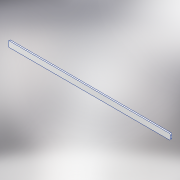
# Autodesk Inventor part: 2021-01-008
Saved by Autodesk Inventor 2020.2 (Build 242310000, 310)
## iProperties
Created: 2020-10-08
Part Number: 2021-01-008
Material: Aluminum 6061
Document SubType Name: Modeling
Designer: carso
Density: 2.7 g/cm^3
Appearance: Aluminum - Flat
Mass: 37.4495 g
Surface Area: 115.086 cm^2
Volume: 13.8702 cm^3
Author: carso
Autodesk Inventor part; units mm, degrees
ref_plane "YZ Plane" through (0, 0, 0) normal (1, 0, 0) x (0, 1, 0)
ref_plane "XZ Plane" through (0, 0, 0) normal (0, 1, 0) x (-1, 0, 0)
ref_plane "XY Plane" through (0, 0, 0) normal (0, 0, 1) x (1, 0, 0)
sketch "Sketch1" plane through (0, 0, 0) normal (0, 0, 1) x (1, 0, 0)
  line L0 (0, -3) -> (349.95, -3)
  line L1 (352.95, -6) -> (352.95, -13.05)
  line L2 (349.95, -16.05) -> (0, -16.05)
  line L3 (-3, -13.05) -> (-3, -6)
  arc A0 (352.95, -6) -> (349.95, -3) centre (349.95, -6) ccw
  arc A1 (349.95, -16.05) -> (352.95, -13.05) centre (349.95, -13.05) ccw
  arc A2 (0, -3) -> (-3, -6) centre (0, -6) ccw
  arc A3 (-3, -13.05) -> (0, -16.05) centre (0, -13.05) ccw
  point P0 (0, 0)
  point P1 (-6, -19.05)
  dimension "d0" = 3
  constraints: 8 end point, 8 point on circle, 8 tangent, 4 centre point, 3 equal radius, 2 parallel, 1 horizontal, 1 perpendicular
  measures "d0" radius of A0
extrude "Extrusion1" add sketch "Sketch1" along normal blind 3
sketch "Sketch2" plane through (0, 0, 3) normal (0, 0, 1) x (1, 0, 0)
  line L0 (-3, -3) -> (352.95, -3)
  line L1 (352.95, -3) -> (352.95, -16.05)
  line L2 (352.95, -16.05) -> (-3, -16.05)
  line L3 (-3, -16.05) -> (-3, -3)
  line L4 (174.975, -9.525) -> (174.975, -13.6338)
  line L5 (33.6, -9.525) -> (316.35, -9.525) construction
  line L6 (33.6, -11.025) -> (316.35, -11.025)
  line L7 (316.35, -8.025) -> (33.6, -8.025)
  arc A0 (33.6, -8.025) -> (33.6, -11.025) centre (33.6, -9.525) ccw
  arc A1 (316.35, -11.025) -> (316.35, -8.025) centre (316.35, -9.525) ccw
  point P0 (0, 0)
  dimension "d4" = 3
  constraints: 18 end point, 4 point on circle, 4 tangent, 3 parallel, 2 centre point, 2 perpendicular, 1 horizontal, 1 midpoint, 1 vertical
  measures "d4" diameter of A1
sketch "Sketch3" plane through (0, 0, 0) normal (0, 0, -1) x (-1, 0, 0)
  line L0 (-352.95, -3) -> (3, -3)
  line L1 (3, -3) -> (3, -16.05)
  line L2 (3, -16.05) -> (-352.95, -16.05)
  line L3 (-352.95, -16.05) -> (-352.95, -3)
  line L4 (0, -16.05) -> (-349.95, -16.05)
  line L5 (-352.95, -3) -> (-322.95, -3)
  line L6 (-322.95, -3) -> (-322.95, -16.05)
  line L7 (-322.95, -16.05) -> (-352.95, -16.05)
  line L8 (-352.95, -16.05) -> (-352.95, -3)
  line L9 (3, -3) -> (-27, -3)
  line L10 (-27, -3) -> (-27, -16.05)
  line L11 (-27, -16.05) -> (3, -16.05)
  line L12 (3, -16.05) -> (3, -3)
  line L13 (-322.95, -3) -> (-322.95, -9.525)
  line L14 (-322.95, -9.525) -> (-27, -9.525)
  line L15 (-322.95, -9.525) -> (-292.95, -9.525)
  line L16 (-27, -9.525) -> (-57, -9.525)
  circle A0 centre (-292.95, -9.525) radius 2.5
  circle A1 centre (-57, -9.525) radius 2.5
  line L17 (-290.45, -9.525) -> (-285.45, -9.525)
  line L18 (-352.95, -3) -> (3, -3)
  line L19 (3, -3) -> (3, -16.05)
  line L20 (3, -16.05) -> (-352.95, -16.05)
  line L21 (-352.95, -16.05) -> (-352.95, -3)
  point P0 (0, 0)
  point P1 (-355.95, -19.05)
  dimension "d7" = 30
  dimension "d8" = 30
  dimension "d9" = 6.525
  dimension "d10" = 30
  dimension "d11" = 30
  dimension "d12" = 5
  dimension "d13" = 5
  constraints: 44 end point, 8 parallel, 6 point on line, 4 horizontal, 4 perpendicular, 2 coincident, 2 midpoint, 1 centre point, 1 horizontal alignment, 2 other
  measures "d7" distance of L6.end L7.end
  measures "d8" distance of L11.end L10.end
  measures "d9" distance of L5.end L13.end
  measures "d10" distance of L13.end L15.end
  measures "d11" distance of L14.end L16.end
  measures "d12" diameter of A1
  measures "d13" distance of L17.start L17.end
extrude "Extrusion3" cut sketch "Sketch3" against normal blind 1 contours A0 L14 | L14 A0 | A1 L14 | L14 A1
sketch "Sketch4" plane through (57, -9.525, 1) normal (0, 0, -1) x (-1, 0, 0)
  circle A0 centre (0, 0) radius 2.5
  circle A1 centre (-235.95, 0) radius 2.5 projected
  circle A2 centre (-235.95, 0) radius 2.5
  circle A3 centre (-235.95, 0) radius 1.5
  circle A4 centre (0, 0) radius 1.5
  point P0 (57, 9.525)
  dimension "d16" = 1
  dimension "d17" = 1
  constraints: 4 centre point, 1 coincident
  measures "d16" radial gap between concentric circles of A1 A3
  measures "d17" radial gap between concentric circles of A0 A4
extrude "Extrusion4" cut sketch "Sketch4" against normal blind 0.2 contours A3 | A4
sketch "Sketch5" plane through (0, 0, 3) normal (0, 0, 1) x (1, 0, 0)
  line L0 (352.95, -13.05) -> (352.95, -6) projected
  arc A0 (352.95, -6) -> (349.95, -3) centre (349.95, -6) ccw projected
  line L1 (349.95, -3) -> (0, -3) projected
  arc A1 (0, -3) -> (-3, -6) centre (0, -6) ccw projected
  line L2 (-3, -6) -> (-3, -13.05) projected
  arc A2 (-3, -13.05) -> (0, -16.05) centre (0, -13.05) ccw projected
  line L3 (0, -16.05) -> (349.95, -16.05) projected
  arc A3 (349.95, -16.05) -> (352.95, -13.05) centre (349.95, -13.05) ccw projected
  line L4 (0, -2.975) -> (349.95, -2.975)
  arc A4 (352.975, -6) -> (349.95, -2.975) centre (349.95, -6) ccw
  line L5 (352.975, -6) -> (352.975, -13.05)
  arc A5 (349.95, -16.075) -> (352.975, -13.05) centre (349.95, -13.05) ccw
  line L6 (349.95, -16.075) -> (0, -16.075)
  arc A6 (-3.025, -13.05) -> (0, -16.075) centre (0, -13.05) ccw
  line L7 (-3.025, -13.05) -> (-3.025, -6)
  arc A7 (0, -2.975) -> (-3.025, -6) centre (0, -6) ccw
  point P0 (0, 0)
  dimension "d20" = 0.025
  constraints: 8 end point, 8 point on circle, 4 centre point, 7 other
  measures "d20" distance between parallel lines of L1 L4
extrude "Extrusion5" add sketch "Sketch5" against normal up to surface (3 mm away)
sketch "Sketch6" plane through (0, 0, 3) normal (0, 0, 1) x (1, 0, 0)
  line L0 (352.975, -13.05) -> (352.975, -6) projected
  arc A0 (352.975, -6) -> (349.95, -2.975) centre (349.95, -6) ccw projected
  line L1 (349.95, -2.975) -> (0, -2.975) projected
  arc A1 (0, -2.975) -> (-3.025, -6) centre (0, -6) ccw projected
  line L2 (-3.025, -6) -> (-3.025, -13.05) projected
  arc A2 (-3.025, -13.05) -> (0, -16.075) centre (0, -13.05) ccw projected
  line L3 (0, -16.075) -> (349.95, -16.075) projected
  arc A3 (349.95, -16.075) -> (352.975, -13.05) centre (349.95, -13.05) ccw projected
  line L4 (0, -3.175) -> (349.95, -3.175)
  arc A4 (352.775, -6) -> (349.95, -3.175) centre (349.95, -6) ccw
  line L5 (352.775, -6) -> (352.775, -13.05)
  arc A5 (349.95, -15.875) -> (352.775, -13.05) centre (349.95, -13.05) ccw
  line L6 (349.95, -15.875) -> (0, -15.875)
  arc A6 (-2.825, -13.05) -> (0, -15.875) centre (0, -13.05) ccw
  line L7 (-2.825, -13.05) -> (-2.825, -6)
  arc A7 (0, -3.175) -> (-2.825, -6) centre (0, -6) ccw
  point P0 (0, 0)
  dimension "d23" = 0.2
  constraints: 8 end point, 8 point on circle, 4 centre point, 7 other
  measures "d23" distance between parallel lines of L1 L4
extrude "Extrusion6" cut sketch "Sketch6" against normal blind 10
sketch "Sketch7" plane through (0, 0, 0) normal (0, 0, -1) x (-1, 0, 0)
  circle A0 centre (-57, -9.525) radius 1.5 projected
  circle A1 centre (-57, -9.525) radius 2.55
  circle A2 centre (-292.95, -9.525) radius 1.5 projected
  circle A3 centre (-292.95, -9.525) radius 2.55
  point P0 (0, 0)
  dimension "d26" = 5.1
  dimension "d27" = 5.1
  constraints: 2 centre point, 2 coincident
  measures "d26" diameter of A1
  measures "d27" diameter of A3
extrude "Extrusion7" cut sketch "Sketch7" against normal up to surface (1 mm away)
body "Solid1"
